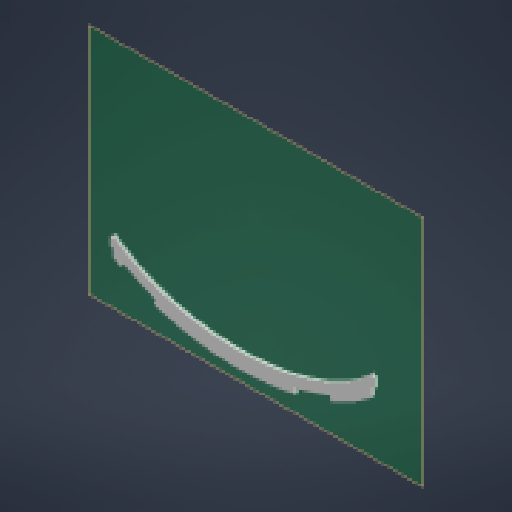
# Autodesk Inventor part: Spant
Saved by Autodesk Inventor 2023 (Build 270158000, 158)
## iProperties
Created: 2022-06-17
Part Number: Spant
Material: Generic
Document SubType Name: Modeling
Designer: bananenbrot
Density: 1 g/cm^3
Appearance: Default
Author: bananenbrot
Autodesk Inventor part; units mm, degrees
ref_plane "YZ Plane" through (0, 0, 0) normal (1, 0, 0) x (0, 1, 0)
ref_plane "XZ Plane" through (0, 0, 0) normal (0, 1, 0) x (-1, 0, 0)
ref_plane "XY Plane" through (0, 0, 0) normal (0, 0, 1) x (1, 0, 0)
ref_plane "Work Plane1" through (0, 0, 0) normal (0, 0, -1) x (-1, 0, 0)
sketch "Sketch1" plane through (0, 0, 0) normal (0, 0, -1) x (-1, 0, 0)
  spline S0 degree 3 poles (105.488254, 71.058726) (105.655909, 71.469411) (105.824043, 71.880004) (106.156862, 72.690396) (106.321597, 73.090375) (106.486681, 73.490119) knots 0 0 0 0 0.50633528 0.50633528 1 1 1 1
  spline S1 degree 3 poles (106.486681, 73.490119) (99.341384, 77.505424) (91.623026, 81.110604) (83.425971, 84.259639) knots -25.89555236 -25.89555236 -25.89555236 -25.89555236 -23.89595958 -23.89595958 -23.89595958 -23.89595958
  spline S2 degree 3 poles (83.425971, 84.259639) (83.383031, 84.186182) (83.340079, 84.112732) (83.249809, 83.958418) (83.202489, 83.877555) (83.155155, 83.796701) knots 0 0 0 0 0.47593748 0.47593748 1 1 1 1
  spline S3 degree 3 poles (83.155155, 83.796701) (82.99498, 83.50339) (82.834647, 83.210135) (82.513677, 82.623784) (82.353014, 82.330641) (82.192209, 82.037607) knots 0 0 0 0 0.49995529 0.49995529 1 1 1 1
  spline S4 degree 3 poles (82.192209, 82.037607) (86.075009, 80.386549) (89.943485, 78.66542) (97.708877, 75.024479) (101.631748, 73.086364) (105.488254, 71.058726) knots -2.57301498 -2.57301498 -2.57301498 -2.57301498 -1.30716712 -1.30716712 -0.00005006 -0.00005006 -0.00005006 -0.00005006
  spline S5 degree 3 poles (-58.922767, -91.941666) (-58.774909, -91.527729) (-58.626707, -91.113855) (-58.3286, -90.283485) (-58.17865, -89.866881) (-58.028364, -89.450461) knots 0 0 0 0 0.49821081 0.49821081 1 1 1 1
  spline S6 degree 3 poles (-58.028364, -89.450461) (-62.223821, -88.294879) (-66.410527, -87.076871) (-74.82943, -84.476914) (-79.083634, -83.084228) (-83.295327, -81.612273) knots -2.64342131 -2.64342131 -2.64342131 -2.64342131 -1.33846844 -1.33846844 -0.00001781 -0.00001781 -0.00001781 -0.00001781
  spline S7 degree 3 poles (-83.295327, -81.612273) (-83.368111, -81.939178) (-83.441155, -82.266061) (-83.587693, -82.919559) (-83.661203, -83.246243) (-83.734938, -83.572841) knots 0 0 0 0 0.50006828 0.50006828 1 1 1 1
  spline S8 degree 3 poles (-83.734938, -83.572841) (-83.752629, -83.665103) (-83.770343, -83.757362) (-83.804214, -83.933539) (-83.820367, -84.01746) (-83.836539, -84.101376) knots 0 0 0 0 0.52364207 0.52364207 1 1 1 1
  spline S9 degree 3 poles (-83.836539, -84.101376) (-75.900663, -87.170821) (-67.564129, -89.792222) (-58.922767, -91.941666) knots -18.70758966 -18.70758966 -18.70758966 -18.70758966 -16.3084011 -16.3084011 -16.3084011 -16.3084011
  spline S10 degree 3 poles (-140.156146, 42.705244) (-140.52655, 42.946666) (-140.896999, 43.188241) (-141.61629, 43.657531) (-141.965329, 43.88536) (-142.314244, 44.113207) knots 0 0 0 0 0.51480121 0.51480121 1 1 1 1
  spline S11 degree 3 poles (-142.314244, 44.113207) (-146.113734, 39.366065) (-149.438319, 34.257689) (-152.104054, 28.810883) knots -4.82793939 -4.82793939 -4.82793939 -4.82793939 -3.00658211 -3.00658211 -3.00658211 -3.00658211
  spline S12 degree 3 poles (-152.104054, 28.810883) (-152.064303, 28.781841) (-152.024554, 28.752797) (-151.909264, 28.668547) (-151.833725, 28.613333) (-151.758195, 28.558111) knots 0 0 0 0 0.344756 0.344756 1 1 1 1
  spline S13 degree 3 poles (-151.758195, 28.558111) (-151.483888, 28.367342) (-151.209569, 28.176431) (-150.661151, 27.794486) (-150.386901, 27.603345) (-150.112796, 27.412158) knots 0 0 0 0 0.49994705 0.49994705 1 1 1 1
  spline S14 degree 3 poles (-150.112796, 27.412158) (-148.553563, 30.128813) (-146.873692, 32.828621) (-143.542191, 37.897752) (-141.864648, 40.324826) (-140.156146, 42.705244) knots -1.81999292 -1.81999292 -1.81999292 -1.81999292 -0.87903361 -0.87903361 -0.00000955 -0.00000955 -0.00000955 -0.00000955
  spline S15 degree 3 poles (-55.772759, -89.028179) (-55.938485, -89.473405) (-56.103756, -89.918878) (-56.433281, -90.809909) (-56.597586, -91.255603) (-56.761424, -91.701392) knots 0 0 0 0 0.50006611 0.50006611 1 1 1 1
  spline S16 degree 3 poles (-56.761424, -91.701392) (-56.698316, -91.71797) (-56.635205, -91.734536) (-56.508995, -91.767635) (-56.445896, -91.784169) (-56.382794, -91.80069) knots 0 0 0 0 0.50007704 0.50007704 1 1 1 1
  spline S17 degree 3 poles (-56.382794, -91.80069) (-56.221993, -91.320035) (-56.060734, -90.839439) (-55.737349, -89.878637) (-55.575164, -89.398259) (-55.412537, -88.918128) knots 0 0 0 0 0.49995781 0.49995781 1 1 1 1
  spline S18 degree 3 poles (-55.412537, -88.918128) (-60.395889, -87.574654) (-65.371777, -86.143235) (-75.376216, -83.050578) (-80.443009, -81.371101) (-85.442136, -79.575514) knots -3.14153253 -3.14153253 -3.14153253 -3.14153253 -1.59354523 -1.59354523 0 0 0 0
  spline S19 degree 3 poles (-85.442136, -79.575514) (-85.600845, -80.347246) (-85.761456, -81.119077) (-86.083068, -82.648175) (-86.244205, -83.406358) (-86.406726, -84.163805) knots 0 0 0 0 0.50422346 0.50422346 1 1 1 1
  spline S20 degree 3 poles (-86.406726, -84.163805) (-90.920076, -82.353793) (-95.299024, -80.397526) (-116.019517, -70.109373) (-129.760695, -59.970512) (-146.159331, -41.459598) (-151.350121, -33.629327) (-158.207877, -17.049282) (-159.996164, -8.655283) (-159.999998, -0.018499) (-160, -0.009249) (-160, 0) knots -11.1695193 -11.1695193 -11.1695193 -11.1695193 -9.98830114 -9.98830114 -5.37837028 -5.37837028 -2.58826084 -2.58826084 0 0 0.00277479 0.00277479 0.00277479 0.00277479
  spline S21 degree 3 poles (-160, 0) (-160, 0.009249) (-159.999998, 0.018499) (-159.996164, 8.655283) (-158.207877, 17.049282) (-154.531773, 25.937027) (-154.137586, 26.837245) (-153.725914, 27.72876) knots -31.82936206 -31.82936206 -31.82936206 -31.82936206 -31.82614588 -31.82614588 -28.82616147 -28.82616147 -28.48444547 -28.48444547 -28.48444547 -28.48444547
  spline S22 degree 3 poles (-153.725914, 27.72876) (-153.133623, 27.312391) (-152.540944, 26.89493) (-151.307606, 26.024278) (-150.664927, 25.569494) (-150.024025, 25.114699) knots 0 0 0 0 0.47946727 0.47946727 1 1 1 1
  spline S23 degree 3 poles (-150.024025, 25.114699) (-148.218657, 28.38678) (-146.211118, 31.651154) (-142.262605, 37.660516) (-140.273177, 40.511906) (-138.247084, 43.294789) knots -2.15697753 -2.15697753 -2.15697753 -2.15697753 -1.03269259 -1.03269259 0 0 0 0
  spline S24 degree 3 poles (-138.247084, 43.294789) (-138.665982, 43.579459) (-139.084954, 43.86436) (-139.922388, 44.434153) (-140.341161, 44.719256) (-140.759707, 45.004364) knots 0 0 0 0 0.50002009 0.50002009 1 1 1 1
  spline S25 degree 3 poles (-140.759707, 45.004364) (-140.786159, 44.968837) (-140.812601, 44.933303) (-140.86548, 44.862206) (-140.891916, 44.826642) (-140.918342, 44.791072) knots 0 0 0 0 0.4998879 0.4998879 1 1 1 1
  spline S26 degree 3 poles (-140.918342, 44.791072) (-140.521169, 44.532497) (-140.123801, 44.273942) (-139.329134, 43.757192) (-138.931577, 43.49883) (-138.534074, 43.240669) knots 0 0 0 0 0.49997548 0.49997548 1 1 1 1
  spline S27 degree 3 poles (-138.534074, 43.240669) (-140.582745, 40.421432) (-142.593714, 37.531617) (-146.438167, 31.657619) (-148.325685, 28.585569) (-150.038777, 25.502731) knots -2.10107116 -2.10107116 -2.10107116 -2.10107116 -1.05805088 -1.05805088 0 0 0 0
  spline S28 degree 3 poles (-150.038777, 25.502731) (-150.450899, 25.794235) (-150.863559, 26.085631) (-151.688414, 26.66721) (-152.101208, 26.957814) (-152.513901, 27.247943) knots 0 0 0 0 0.50015658 0.50015658 1 1 1 1
  spline S29 degree 3 poles (-152.513901, 27.247943) (-152.715187, 27.396775) (-152.916565, 27.545554) (-153.272825, 27.808558) (-153.42774, 27.922853) (-153.582675, 28.037097) knots 0 0 0 0 0.56531165 0.56531165 1 1 1 1
  spline S30 degree 3 poles (-153.582675, 28.037097) (-150.112252, 35.463041) (-145.430604, 42.282192) (-129.760695, 59.970512) (-116.019517, 70.109373) (-76.168856, 89.89605) (-48.159301, 97.168531) (10.323594, 101.429176) (40.306692, 98.637427) (72.686621, 89.145496) (77.300324, 87.615382) (81.772002, 85.953611) knots -28.44500583 -28.44500583 -28.44500583 -28.44500583 -25.59221971 -25.59221971 -20.24897129 -20.24897129 -12.68266849 -12.68266849 -5.31702533 -5.31702533 -4.05257189 -4.05257189 -4.05257189 -4.05257189
  spline S31 degree 3 poles (81.772002, 85.953611) (81.39685, 85.277236) (81.020675, 84.601078) (80.260988, 83.24002) (79.877131, 82.554568) (79.4924, 81.86999) knots 0 0 0 0 0.49620458 0.49620458 1 1 1 1
  spline S32 degree 3 poles (79.4924, 81.86999) (84.106097, 79.944142) (88.704811, 77.920177) (97.92698, 73.597565) (102.596521, 71.267421) (107.162032, 68.805956) knots -3.05655345 -3.05655345 -3.05655345 -3.05655345 -1.55603451 -1.55603451 0 0 0 0
  spline S33 degree 3 poles (107.162032, 68.805956) (107.362525, 69.272925) (107.563697, 69.739771) (107.967009, 70.672511) (108.169269, 71.138686) (108.372016, 71.604484) knots 0 0 0 0 0.50008693 0.50008693 1 1 1 1
  spline S34 degree 3 poles (108.372016, 71.604484) (108.311413, 71.637617) (108.250793, 71.670727) (108.129563, 71.736879) (108.068966, 71.769912) (108.008356, 71.802922) knots 0 0 0 0 0.50026413 0.50026413 1 1 1 1
  spline S35 degree 3 poles (108.008356, 71.802922) (107.831652, 71.360531) (107.655471, 70.9178) (107.304315, 70.031863) (107.129254, 69.588442) (106.954875, 69.144881) knots 0 0 0 0 0.49987396 0.49987396 1 1 1 1
  spline S36 degree 3 poles (106.954875, 69.144881) (102.458096, 71.560882) (97.862015, 73.850273) (88.857802, 78.067945) (84.40815, 80.029312) (79.943507, 81.898722) knots -2.98266168 -2.98266168 -2.98266168 -2.98266168 -1.45206607 -1.45206607 0 0 0 0
  spline S37 degree 3 poles (79.943507, 81.898722) (80.189868, 82.338832) (80.435857, 82.779254) (80.926861, 83.660218) (81.171962, 84.100915) (81.416641, 84.541745) knots 0 0 0 0 0.50009335 0.50009335 1 1 1 1
  spline S38 degree 3 poles (81.416641, 84.541745) (81.544597, 84.757023) (81.672451, 84.972373) (81.922458, 85.393942) (82.044631, 85.600173) (82.166704, 85.806452) knots 0 0 0 0 0.51095751 0.51095751 1 1 1 1
  spline S39 degree 3 poles (82.166704, 85.806452) (96.340132, 80.504804) (109.079769, 73.882769) (120, 66.143783) knots -4.01533339 -4.01533339 -4.01533339 -4.01533339 0 0 0 0
  line L0 (120, 66.143783) -> (120, 64.915839)
  spline S40 degree 3 poles (120, 64.915839) (116.958046, 67.095767) (113.769602, 69.18832) (110.4451, 71.188412) knots -27.23016157 -27.23016157 -27.23016157 -27.23016157 -26.27049987 -26.27049987 -26.27049987 -26.27049987
  spline S41 degree 3 poles (110.4451, 71.188412) (110.144531, 70.479272) (109.845231, 69.769024) (109.241462, 68.327114) (108.936634, 67.594325) (108.633933, 66.86133) knots 0 0 0 0 0.49269339 0.49269339 1 1 1 1
  spline S42 degree 3 poles (108.633933, 66.86133) (103.413337, 69.741468) (98.040638, 72.443923) (87.569561, 77.343921) (82.406444, 79.594098) (77.229578, 81.721673) knots -3.46782142 -3.46782142 -3.46782142 -3.46782142 -1.67911103 -1.67911103 -0.00000822 -0.00000822 -0.00000822 -0.00000822
  spline S43 degree 3 poles (77.229578, 81.721673) (77.614353, 82.392714) (77.998129, 83.064688) (78.756084, 84.39678) (79.130603, 85.057404) (79.504014, 85.718327) knots 0 0 0 0 0.5047033 0.5047033 1 1 1 1
  spline S44 degree 3 poles (79.504014, 85.718327) (76.000382, 86.979279) (72.415021, 88.158572) (41.411665, 97.427275) (11.712347, 100.344863) (-46.584978, 96.460454) (-74.708327, 89.33117) (-114.784395, 69.723313) (-128.606876, 59.635414) (-139.39681, 47.589468) (-139.920365, 46.990667) (-140.436318, 46.385633) knots -23.57993789 -23.57993789 -23.57993789 -23.57993789 -22.74051364 -22.74051364 -16.46951252 -16.46951252 -9.96116021 -9.96116021 -5.36021524 -5.36021524 -5.12219462 -5.12219462 -5.12219462 -5.12219462
  spline S45 degree 3 poles (-140.436318, 46.385633) (-139.821337, 45.967601) (-139.205726, 45.549511) (-137.937927, 44.689331) (-137.284591, 44.246513) (-136.631622, 43.804456) knots 0 0 0 0 0.48532424 0.48532424 1 1 1 1
  spline S46 degree 3 poles (-136.631622, 43.804456) (-139.054316, 40.516338) (-141.435007, 37.123701) (-145.886157, 30.29577) (-148.055837, 26.710869) (-149.950671, 23.137939) knots -2.43253078 -2.43253078 -2.43253078 -2.43253078 -1.21332259 -1.21332259 -0.00004072 -0.00004072 -0.00004072 -0.00004072
  spline S47 degree 3 poles (-149.950671, 23.137939) (-150.579311, 23.592648) (-151.210164, 24.04715) (-152.403565, 24.90403) (-152.968317, 25.308301) (-153.532797, 25.711303) knots 0 0 0 0 0.52806556 0.52806556 1 1 1 1
  spline S48 degree 3 poles (-153.532797, 25.711303) (-153.653765, 25.431767) (-153.772984, 25.151387) (-157.199149, 16.9475) (-158.99615, 8.606573) (-158.999998, 0.018371) (-159, 0.009185) (-159, 0) knots -2.66506067 -2.66506067 -2.66506067 -2.66506067 -2.57370536 -2.57370536 0 0 0.00275564 0.00275564 0.00275564 0.00275564
  spline S49 degree 3 poles (-159, 0) (-159, -0.009185) (-158.999998, -0.018371) (-158.99615, -8.606573) (-157.199149, -16.9475) (-150.308131, -33.447912) (-145.079436, -41.245352) (-128.606876, -59.635414) (-114.784395, -69.723313) (-94.929583, -79.437598) (-91.582833, -80.947001) (-88.154881, -82.370355) knots -31.86013737 -31.86013737 -31.86013737 -31.86013737 -31.85691351 -31.85691351 -28.84590276 -28.84590276 -25.5859293 -25.5859293 -20.20322506 -20.20322506 -19.14689485 -19.14689485 -19.14689485 -19.14689485
  spline S50 degree 3 poles (-88.154881, -82.370355) (-88.005245, -81.625565) (-87.857245, -80.880017) (-87.561724, -79.371575) (-87.414116, -78.607759) (-87.268731, -77.844009) knots 0 0 0 0 0.49421065 0.49421065 1 1 1 1
  spline S51 degree 3 poles (-87.268731, -77.844009) (-81.548725, -79.948527) (-75.730398, -81.89586) (-64.370585, -85.404573) (-58.77266, -86.997837) (-53.169946, -88.480229) knots -3.56732869 -3.56732869 -3.56732869 -3.56732869 -1.7386564 -1.7386564 -0.00000461 -0.00000461 -0.00000461 -0.00000461
  spline S52 degree 3 poles (-53.169946, -88.480229) (-53.431004, -89.225816) (-53.690828, -89.9722) (-54.206068, -91.460346) (-54.461722, -92.202741) (-54.716118, -92.945222) knots 0 0 0 0 0.50162275 0.50162275 1 1 1 1
  spline S53 degree 3 poles (-54.716118, -92.945222) (-42.581047, -95.718052) (-29.888292, -97.572971) (11.712347, -100.344863) (41.411665, -97.427275) (88.330972, -83.40037) (105.768628, -75.114337) (120, -64.915839) knots -15.92125118 -15.92125118 -15.92125118 -15.92125118 -12.58902064 -12.58902064 -5.2524964 -5.2524964 0 0 0 0
  line L1 (120, -64.915839) -> (120, -66.143783)
  spline S54 degree 3 poles (120, -66.143783) (105.539645, -76.391596) (87.891779, -84.688219) (40.306692, -98.637427) (10.323594, -101.429176) (-42.625257, -97.571702) (-65.649403, -92.429988) (-85.972732, -84.337236) knots -27.4582651 -27.4582651 -27.4582651 -27.4582651 -22.87095843 -22.87095843 -16.51619015 -16.51619015 -11.20734468 -11.20734468 -11.20734468 -11.20734468
  spline S55 degree 3 poles (-85.972732, -84.337236) (-85.929472, -84.101334) (-85.886373, -83.86539) (-85.798444, -83.382085) (-85.753625, -83.134694) (-85.708998, -82.887282) knots 0 0 0 0 0.488224 0.488224 1 1 1 1
  spline S56 degree 3 poles (-85.708998, -82.887282) (-85.603052, -82.392867) (-85.49772, -81.898193) (-85.288395, -80.908503) (-85.184351, -80.41324) (-85.081049, -79.917953) knots 0 0 0 0 0.49984979 0.49984979 1 1 1 1
  spline S57 degree 3 poles (-85.081049, -79.917953) (-80.168058, -81.674386) (-75.190842, -83.31947) (-65.425689, -86.333614) (-60.603113, -87.722189) (-55.772759, -89.028179) knots -3.06681768 -3.06681768 -3.06681768 -3.06681768 -1.50113749 -1.50113749 0 0 0 0
  line L2 (-130, 140) -> (-130, -140)
  ellipse E0 centre (0, 0) end of major axis (0, -84.000351) minor radius 144 (-130, -36.129164) -> (120, -46.432941) ccw
  line L3 (120, -64.915839) -> (120, -46.432941)
  spline S58 degree 3 poles (83.155155, -83.796701) (83.202489, -83.877556) (83.24981, -83.958419) (83.340079, -84.112732) (83.383031, -84.186182) (83.425971, -84.259639) knots 0 0 0 0 0.52406443 0.52406443 1 1 1 1
  spline S59 degree 3 poles (83.425971, -84.259639) (91.623023, -81.110605) (99.341382, -77.505425) (106.486681, -73.490119) knots -3.90072545 -3.90072545 -3.90072545 -3.90072545 -1.56137635 -1.56137635 -1.56137635 -1.56137635
  spline S60 degree 3 poles (106.486681, -73.490119) (106.321618, -73.090425) (106.156903, -72.690495) (105.824083, -71.880103) (105.655929, -71.469461) (105.488254, -71.058726) knots 0 0 0 0 0.49360341 0.49360341 1 1 1 1
  spline S61 degree 3 poles (105.488254, -71.058726) (101.601392, -73.102325) (97.647003, -75.055044) (89.880457, -78.693455) (86.043436, -80.399975) (82.192209, -82.037607) knots -2.57282162 -2.57282162 -2.57282162 -2.57282162 -1.25548991 -1.25548991 -0.00000561 -0.00000561 -0.00000561 -0.00000561
  spline S62 degree 3 poles (82.192209, -82.037607) (82.353014, -82.330641) (82.513677, -82.623785) (82.834648, -83.210136) (82.99498, -83.50339) (83.155155, -83.796701) knots 0 0 0 0 0.50004508 0.50004508 1 1 1 1
  spline S63 degree 3 poles (-58.028364, -89.450461) (-62.233064, -88.292333) (-66.429007, -87.071495) (-74.847725, -84.470924) (-79.092678, -83.081067) (-83.295327, -81.612273) knots -2.64341286 -2.64341286 -2.64341286 -2.64341286 -1.33558505 -1.33558505 -0.00000826 -0.00000826 -0.00000826 -0.00000826
  spline S64 degree 3 poles (-83.295327, -81.612273) (-83.368111, -81.939178) (-83.441155, -82.266061) (-83.587693, -82.91956) (-83.661203, -83.246244) (-83.734938, -83.572841) knots 0 0 0 0 0.50006844 0.50006844 1 1 1 1
  spline S65 degree 3 poles (-83.734938, -83.572841) (-83.752651, -83.665214) (-83.770386, -83.757584) (-83.804257, -83.933762) (-83.820388, -84.017571) (-83.836539, -84.101376) knots 0 0 0 0 0.52427325 0.52427325 1 1 1 1
  spline S66 degree 3 poles (-83.836539, -84.101376) (-77.593042, -86.516243) (-71.077682, -88.662135) (-64.355901, -90.51692) (-62.559229, -91.012688) (-60.747638, -91.487388) (-58.922767, -91.941666) knots 0 0 0 0 0.78908463 0.78908463 0.78908463 1 1 1 1
  spline S67 degree 3 poles (-58.922767, -91.941666) (-58.774903, -91.527713) (-58.626695, -91.113822) (-58.328588, -90.283452) (-58.178644, -89.866865) (-58.028364, -89.450461) knots 0 0 0 0 0.49823074 0.49823074 1 1 1 1
  spline S68 degree 3 poles (82.192209, 82.037607) (86.086099, 80.381833) (89.965626, 78.655569) (97.730611, 75.013739) (101.642413, 73.080757) (105.488254, 71.058726) knots -2.57298365 -2.57298365 -2.57298365 -2.57298365 -1.3035202 -1.3035202 -0.00001762 -0.00001762 -0.00001762 -0.00001762
  spline S69 degree 3 poles (105.488254, 71.058726) (105.65593, 71.469462) (105.824085, 71.880106) (106.156904, 72.690498) (106.321618, 73.090426) (106.486681, 73.490119) knots 0 0 0 0 0.50639849 0.50639849 1 1 1 1
  spline S70 degree 3 poles (106.486681, 73.490119) (99.336447, 77.508199) (91.617269, 81.112815) (83.425971, 84.259639) knots -20.48335777 -20.48335777 -20.48335777 -20.48335777 -18.34027175 -18.34027175 -18.34027175 -18.34027175
  spline S71 degree 3 poles (83.425971, 84.259639) (83.383031, 84.186182) (83.340079, 84.112732) (83.249809, 83.958418) (83.202489, 83.877555) (83.155155, 83.796701) knots 0 0 0 0 0.4759375 0.4759375 1 1 1 1
  spline S72 degree 3 poles (83.155155, 83.796701) (82.99498, 83.50339) (82.834647, 83.210135) (82.513677, 82.623784) (82.353014, 82.330641) (82.192209, 82.037607) knots 0 0 0 0 0.49995542 0.49995542 1 1 1 1
  spline S73 degree 3 poles (-83.295327, 81.612273) (-79.056214, 83.093811) (-74.773955, 84.495073) (-66.354492, 87.093168) (-62.195794, 88.302599) (-58.028364, 89.450461) knots -2.64454735 -2.64454735 -2.64454735 -2.64454735 -1.29681005 -1.29681005 -0.00002349 -0.00002349 -0.00002349 -0.00002349
  spline S74 degree 3 poles (-58.028364, 89.450461) (-58.178669, 89.866933) (-58.328637, 90.283589) (-58.626744, 91.113959) (-58.774927, 91.527781) (-58.922767, 91.941666) knots 0 0 0 0 0.50185207 0.50185207 1 1 1 1
  spline S75 degree 3 poles (-58.922767, 91.941666) (-67.552935, 89.794994) (-75.890466, 87.174767) (-83.836539, 84.101376) knots -7.08866348 -7.08866348 -7.08866348 -7.08866348 -4.92689897 -4.92689897 -4.92689897 -4.92689897
  spline S76 degree 3 poles (-83.836539, 84.101376) (-83.820367, 84.01746) (-83.804214, 83.93354) (-83.770343, 83.757363) (-83.752629, 83.665103) (-83.734938, 83.572841) knots 0 0 0 0 0.47635613 0.47635613 1 1 1 1
  spline S77 degree 3 poles (-83.734938, 83.572841) (-83.661203, 83.246243) (-83.587693, 82.919559) (-83.441155, 82.26606) (-83.368111, 81.939178) (-83.295327, 81.612273) knots 0 0 0 0 0.49993221 0.49993221 1 1 1 1
  spline S78 degree 3 poles (120, 64.915839) (116.957002, 67.096515) (113.76848, 69.188995) (110.4451, 71.188412) knots -21.91218991 -21.91218991 -21.91218991 -21.91218991 -20.88499187 -20.88499187 -20.88499187 -20.88499187
  spline S79 degree 3 poles (110.4451, 71.188412) (110.14453, 70.479268) (109.845229, 69.769017) (109.241459, 68.327108) (108.936633, 67.594322) (108.633933, 66.86133) knots 0 0 0 0 0.49269556 0.49269556 1 1 1 1
  spline S80 degree 3 poles (108.633933, 66.86133) (103.399335, 69.749193) (98.011719, 72.458471) (87.539917, 77.356836) (82.391633, 79.600185) (77.229578, 81.721673) knots -3.46781506 -3.46781506 -3.46781506 -3.46781506 -1.67430729 -1.67430729 -0.00000822 -0.00000822 -0.00000822 -0.00000822
  spline S81 degree 3 poles (77.229578, 81.721673) (77.614354, 82.392716) (77.998131, 83.064691) (78.756086, 84.396783) (79.130604, 85.057405) (79.504014, 85.718327) knots 0 0 0 0 0.5047044 0.5047044 1 1 1 1
  spline S82 degree 3 poles (79.504014, 85.718327) (73.308954, 87.94792) (66.861755, 89.921003) (36.694093, 97.614716) (11.758891, 99.889296) (-27.015369, 97.977443) (-41.19803, 96.03407) (-54.716118, 92.945222) knots -18.00144011 -18.00144011 -18.00144011 -18.00144011 -16.40919862 -16.40919862 -10.78869968 -10.78869968 -7.43834932 -7.43834932 -7.43834932 -7.43834932
  spline S83 degree 3 poles (-54.716118, 92.945222) (-54.461721, 92.202737) (-54.206066, 91.460338) (-53.690825, 89.972192) (-53.431002, 89.225812) (-53.169946, 88.480229) knots 0 0 0 0 0.49837992 0.49837992 1 1 1 1
  spline S84 degree 3 poles (-53.169946, 88.480229) (-58.845945, 86.978447) (-64.517386, 85.362779) (-75.875221, 81.847348) (-81.619734, 79.922402) (-87.268731, 77.844009) knots -3.5669406 -3.5669406 -3.5669406 -3.5669406 -1.80576616 -1.80576616 -0.00000315 -0.00000315 -0.00000315 -0.00000315
  spline S85 degree 3 poles (-87.268731, 77.844009) (-87.414117, 78.607768) (-87.561728, 79.371592) (-87.857248, 80.880034) (-88.005246, 81.625573) (-88.154881, 82.370355) knots 0 0 0 0 0.50579491 0.50579491 1 1 1 1
  spline S86 degree 3 poles (-88.154881, 82.370355) (-104.503687, 75.582004) (-118.684509, 66.972452) (-130, 56.965589) knots -4.53204805 -4.53204805 -4.53204805 -4.53204805 -0.00045691 -0.00045691 -0.00045691 -0.00045691
  line L4 (-130, 56.965589) -> (-130, 58.296119)
  spline S87 degree 3 poles (-130, 58.296119) (-118.207585, 68.568391) (-103.411704, 77.344214) (-86.406726, 84.163805) knots -23.34438249 -23.34438249 -23.34438249 -23.34438249 -18.59383478 -18.59383478 -18.59383478 -18.59383478
  spline S88 degree 3 poles (-86.406726, 84.163805) (-86.244204, 83.406352) (-86.083065, 82.648162) (-85.761453, 81.119064) (-85.600844, 80.347239) (-85.442136, 79.575514) knots 0 0 0 0 0.49578079 0.49578079 1 1 1 1
  spline S89 degree 3 poles (-85.442136, 79.575514) (-80.397499, 81.387447) (-75.283769, 83.081215) (-65.278219, 86.170137) (-60.349134, 87.587259) (-55.412537, 88.918128) knots -3.14230865 -3.14230865 -3.14230865 -3.14230865 -1.53385404 -1.53385404 0 0 0 0
  spline S90 degree 3 poles (-55.412537, 88.918128) (-55.575164, 89.39826) (-55.737349, 89.878639) (-56.060735, 90.839441) (-56.221993, 91.320036) (-56.382794, 91.80069) knots 0 0 0 0 0.50004299 0.50004299 1 1 1 1
  spline S91 degree 3 poles (-56.382794, 91.80069) (-56.445896, 91.784169) (-56.508995, 91.767635) (-56.635205, 91.734536) (-56.698317, 91.71797) (-56.761424, 91.701392) knots 0 0 0 0 0.49992367 0.49992367 1 1 1 1
  spline S92 degree 3 poles (-56.761424, 91.701392) (-56.597585, 91.255602) (-56.43328, 90.809907) (-56.103755, 89.918876) (-55.938485, 89.473404) (-55.772759, 89.028179) knots 0 0 0 0 0.49993492 0.49993492 1 1 1 1
  spline S93 degree 3 poles (-55.772759, 89.028179) (-60.650289, 87.709433) (-65.520078, 86.306431) (-75.284135, 83.288618) (-80.214017, 81.657955) (-85.081049, 79.917953) knots -3.06599686 -3.06599686 -3.06599686 -3.06599686 -1.55061421 -1.55061421 0 0 0 0
  spline S94 degree 3 poles (-85.081049, 79.917953) (-85.184352, 80.413241) (-85.288396, 80.908506) (-85.49772, 81.898196) (-85.603052, 82.392868) (-85.708998, 82.887282) knots 0 0 0 0 0.50015183 0.50015183 1 1 1 1
  spline S95 degree 3 poles (-85.708998, 82.887282) (-85.753625, 83.134694) (-85.798444, 83.382086) (-85.886373, 83.865391) (-85.929472, 84.101334) (-85.972732, 84.337236) knots 0 0 0 0 0.51177654 0.51177654 1 1 1 1
  spline S96 degree 3 poles (-85.972732, 84.337236) (-84.39827, 84.964186) (-82.805012, 85.574409) (-61.249176, 93.508605) (-39.799713, 97.77755) (10.323594, 101.429176) (40.306692, 98.637427) (72.686621, 89.145496) (77.300324, 87.615382) (81.772002, 85.953611) knots -18.55346544 -18.55346544 -18.55346544 -18.55346544 -18.11458791 -18.11458791 -12.68266849 -12.68266849 -5.31702533 -5.31702533 -4.05257189 -4.05257189 -4.05257189 -4.05257189
  spline S97 degree 3 poles (81.772002, 85.953611) (81.396849, 85.277235) (81.020673, 84.601075) (80.260986, 83.240017) (79.87713, 82.554567) (79.4924, 81.86999) knots 0 0 0 0 0.49620556 0.49620556 1 1 1 1
  spline S98 degree 3 poles (79.4924, 81.86999) (84.123686, 79.9368) (88.73997, 77.904703) (97.961374, 73.580395) (102.613292, 71.258379) (107.162032, 68.805956) knots -3.05655776 -3.05655776 -3.05655776 -3.05655776 -1.55031837 -1.55031837 0 0 0 0
  spline S99 degree 3 poles (107.162032, 68.805956) (107.362525, 69.272925) (107.563698, 69.739772) (107.967009, 70.672512) (108.169269, 71.138686) (108.372016, 71.604484) knots 0 0 0 0 0.50008746 0.50008746 1 1 1 1
  spline S100 degree 3 poles (108.372016, 71.604484) (108.311413, 71.637617) (108.250793, 71.670727) (108.129563, 71.736879) (108.068966, 71.769913) (108.008356, 71.802922) knots 0 0 0 0 0.50026455 0.50026455 1 1 1 1
  spline S101 degree 3 poles (108.008356, 71.802922) (107.831651, 71.360531) (107.655471, 70.917799) (107.304314, 70.031862) (107.129254, 69.588442) (106.954875, 69.144881) knots 0 0 0 0 0.49987468 0.49987468 1 1 1 1
  spline S102 degree 3 poles (106.954875, 69.144881) (102.448301, 71.566144) (97.841942, 73.860273) (88.837298, 78.076982) (84.397889, 80.033608) (79.943507, 81.898722) knots -2.98265816 -2.98265816 -2.98265816 -2.98265816 -1.44872878 -1.44872878 0 0 0 0
  spline S103 degree 3 poles (79.943507, 81.898722) (80.189868, 82.338833) (80.435857, 82.779254) (80.926861, 83.660218) (81.171962, 84.100915) (81.416641, 84.541745) knots 0 0 0 0 0.5000937 0.5000937 1 1 1 1
  spline S104 degree 3 poles (81.416641, 84.541745) (81.544597, 84.757023) (81.672451, 84.972373) (81.922459, 85.393942) (82.044631, 85.600173) (82.166704, 85.806452) knots 0 0 0 0 0.51095765 0.51095765 1 1 1 1
  spline S105 degree 3 poles (82.166704, 85.806452) (96.340127, 80.504806) (109.079769, 73.882769) (120, 66.143783) knots -4.01533339 -4.01533339 -4.01533339 -4.01533339 0 0 0 0
  line L5 (120, 66.143783) -> (120, 64.915839)
  spline S106 degree 3 poles (-56.761424, -91.701392) (-56.698316, -91.717971) (-56.635205, -91.734536) (-56.508995, -91.767635) (-56.445896, -91.784169) (-56.382794, -91.80069) knots 0 0 0 0 0.50007725 0.50007725 1 1 1 1
  spline S107 degree 3 poles (-56.382794, -91.80069) (-56.221993, -91.320035) (-56.060734, -90.839439) (-55.737349, -89.878637) (-55.575164, -89.398259) (-55.412537, -88.918128) knots 0 0 0 0 0.49995803 0.49995803 1 1 1 1
  spline S108 degree 3 poles (-55.412537, -88.918128) (-60.410207, -87.570794) (-65.400429, -86.134993) (-75.404526, -83.041192) (-80.456947, -81.366095) (-85.442136, -79.575514) knots -3.14153527 -3.14153527 -3.14153527 -3.14153527 -1.58910232 -1.58910232 0 0 0 0
  spline S109 degree 3 poles (-85.442136, -79.575514) (-85.600846, -80.347247) (-85.761456, -81.119081) (-86.083069, -82.648179) (-86.244206, -83.40636) (-86.406726, -84.163805) knots 0 0 0 0 0.50422465 0.50422465 1 1 1 1
  ellipse E1 centre (0, 0) end of major axis (160, 0) minor radius 100 (-130, -58.296119) -> (-86.406726, -84.163805) ccw
  line L6 (-130, -58.296119) -> (-130, -56.965589)
  spline S110 degree 3 poles (-130, -56.965589) (-125.622291, -60.837019) (-120.7953, -64.515531) (-115.568661, -67.961571) (-107.344581, -73.38389) (-98.127989, -78.229321) (-88.154881, -82.370355) knots 0 0 0 0 0.38857691 0.38857691 0.38857691 1 1 1 1
  spline S111 degree 3 poles (-88.154881, -82.370355) (-88.005261, -81.625648) (-87.857277, -80.880183) (-87.561756, -79.371741) (-87.414132, -78.607842) (-87.268731, -77.844009) knots 0 0 0 0 0.49415576 0.49415576 1 1 1 1
  spline S112 degree 3 poles (-87.268731, -77.844009) (-81.53492, -79.953606) (-75.702237, -81.905287) (-64.342042, -85.412695) (-58.758411, -87.001607) (-53.169946, -88.480229) knots -3.56731676 -3.56731676 -3.56731676 -3.56731676 -1.73423435 -1.73423435 -0.00000461 -0.00000461 -0.00000461 -0.00000461
  spline S113 degree 3 poles (-53.169946, -88.480229) (-53.431002, -89.22581) (-53.690824, -89.972189) (-54.206064, -91.460335) (-54.46172, -92.202735) (-54.716118, -92.945222) knots 0 0 0 0 0.50161891 0.50161891 1 1 1 1
  spline S114 degree 3 poles (-54.716118, -92.945222) (-37.103886, -96.969571) (-18.340613, -99.030517) (0.419495, -98.999655) (23.518657, -98.961655) (46.590543, -95.73532) (67.499159, -89.624011) (71.587609, -88.429012) (75.592712, -87.124235) (79.504014, -85.718327) knots -1.92129687 -1.92129687 -1.92129687 -1.92129687 -1.5681642 -1.5681642 -1.5681642 -1.13335493 -1.13335493 -1.13335493 -1.04833277 -1.04833277 -1.04833277 -1.04833277
  spline S115 degree 3 poles (79.504014, -85.718327) (79.130601, -85.057399) (78.756078, -84.39677) (77.998123, -83.064678) (77.61435, -82.392709) (77.229578, -81.721673) knots 0 0 0 0 0.49530047 0.49530047 1 1 1 1
  spline S116 degree 3 poles (77.229578, -81.721673) (82.493633, -79.558265) (87.744095, -77.267835) (98.210861, -72.358213) (103.495791, -69.695979) (108.633933, -66.86133) knots -3.46785791 -3.46785791 -3.46785791 -3.46785791 -1.76047655 -1.76047655 -0.00001749 -0.00001749 -0.00001749 -0.00001749
  spline S117 degree 3 poles (108.633933, -66.86133) (108.936639, -67.594336) (109.24147, -68.327135) (109.84524, -69.769045) (110.144536, -70.479282) (110.4451, -71.188412) knots 0 0 0 0 0.50731401 0.50731401 1 1 1 1
  spline S118 degree 3 poles (110.4451, -71.188412) (113.769602, -69.18832) (116.958046, -67.095767) (120, -64.915839) knots -1.12272047 -1.12272047 -1.12272047 -1.12272047 0 0 0 0
  line L7 (120, -64.915839) -> (120, -66.143783)
  spline S119 degree 3 poles (120, -66.143783) (109.056689, -73.899126) (96.285436, -80.525263) (82.166705, -85.806452) knots -21.95297363 -21.95297363 -21.95297363 -21.95297363 -18.27712891 -18.27712891 -18.27712891 -18.27712891
  spline S120 degree 3 poles (82.166705, -85.806452) (82.044631, -85.600172) (81.922458, -85.393942) (81.672451, -84.972373) (81.544597, -84.757023) (81.416641, -84.541745) knots 0 0 0 0 0.48904289 0.48904289 1 1 1 1
  spline S121 degree 3 poles (81.416641, -84.541745) (81.171961, -84.100914) (80.92686, -83.660215) (80.435856, -82.779252) (80.189868, -82.338831) (79.943507, -81.898722) knots 0 0 0 0 0.49990784 0.49990784 1 1 1 1
  spline S122 degree 3 poles (79.943507, -81.898722) (84.46361, -80.00609) (88.968632, -78.019084) (97.970501, -73.796201) (102.511041, -71.532436) (106.954875, -69.144881) knots -2.98427203 -2.98427203 -2.98427203 -2.98427203 -1.51338261 -1.51338261 0 0 0 0
  spline S123 degree 3 poles (106.954875, -69.144881) (107.129255, -69.588445) (107.304316, -70.031867) (107.655473, -70.917805) (107.831653, -71.360534) (108.008356, -71.802922) knots 0 0 0 0 0.50012853 0.50012853 1 1 1 1
  spline S124 degree 3 poles (108.008356, -71.802922) (108.068966, -71.769912) (108.129563, -71.736878) (108.250794, -71.670727) (108.311413, -71.637617) (108.372016, -71.604484) knots 0 0 0 0 0.49973733 0.49973733 1 1 1 1
  spline S125 degree 3 poles (108.372016, -71.604484) (108.169268, -71.138684) (107.967007, -70.672507) (107.563696, -69.739767) (107.362524, -69.272923) (107.162032, -68.805956) knots 0 0 0 0 0.49991524 0.49991524 1 1 1 1
  spline S126 degree 3 poles (107.162032, -68.805956) (102.546098, -71.294606) (97.823548, -73.649166) (88.599094, -77.966684) (84.053207, -79.96622) (79.4924, -81.86999) knots -3.05517932 -3.05517932 -3.05517932 -3.05517932 -1.48265878 -1.48265878 0 0 0 0
  spline S127 degree 3 poles (79.4924, -81.86999) (79.877133, -82.554572) (80.260992, -83.240027) (81.020679, -84.601086) (81.396852, -85.27724) (81.772002, -85.953611) knots 0 0 0 0 0.50379827 0.50379827 1 1 1 1
  ellipse E2 centre (0, 0) end of major axis (160, 0) minor radius 100 (-85.972732, -84.337236) -> (81.772002, -85.953611) ccw
  spline S128 degree 3 poles (-85.972732, -84.337236) (-85.929472, -84.101334) (-85.886373, -83.86539) (-85.798444, -83.382085) (-85.753625, -83.134694) (-85.708998, -82.887282) knots 0 0 0 0 0.48822419 0.48822419 1 1 1 1
  spline S129 degree 3 poles (-85.708998, -82.887282) (-85.603052, -82.392866) (-85.49772, -81.898192) (-85.288395, -80.908502) (-85.184351, -80.413239) (-85.081049, -79.917953) knots 0 0 0 0 0.49985033 0.49985033 1 1 1 1
  spline S130 degree 3 poles (-85.081049, -79.917953) (-80.15855, -81.677785) (-75.171541, -83.32585) (-65.406162, -86.339235) (-60.593352, -87.724828) (-55.772759, -89.028179) knots -3.06681307 -3.06681307 -3.06681307 -3.06681307 -1.49810422 -1.49810422 0 0 0 0
  spline S131 degree 3 poles (-55.772759, -89.028179) (-55.938485, -89.473405) (-56.103756, -89.918878) (-56.433281, -90.80991) (-56.597586, -91.255603) (-56.761424, -91.701392) knots 0 0 0 0 0.50006637 0.50006637 1 1 1 1
  point P0 (-144, 0)
  point P1 (0.001352, -84.000351)
  point P2 (0.001352, -99.000351)
  point P3 (-130, -56.96558)
  point P4 (-130, -56.965589)
  point P5 (110.445093, -71.188396)
  dimension "d0" = 15
  dimension "d1" = 15
  constraints: 16 end point, 8 vertical, 1 coincident, 1 horizontal alignment, 1 point on line, 1 vertical alignment, 506 other
  measures "d0" distance of point (-159, 0) point (-144, 0)
  measures "d1" distance of point (0.001, -84) point (0.001, -99)
sketch "Sketch1 outline for Extrusion1" plane through (0, 0, 0) normal (0, 0, -1) x (-1, 0, 0)
  spline S0 degree 2 poles (-130, -36.129164) (-20.600041, -170.07827) (120, -46.432941) knots 0 0 0 1 1 1 weights 1 0.49266415 1
  line L0 (120, -64.915839) -> (120, -46.432941)
  spline S1 degree 3 poles (110.445093, -71.188396) (113.769601, -69.188315) (116.958047, -67.095767) (120, -64.915839) knots 0 0 0 0 1 1 1 1
  spline S2 degree 3 poles (108.633933, -66.86133) (108.936639, -67.594336) (109.24147, -68.327135) (109.845238, -69.76904) (110.144531, -70.479271) (110.445093, -71.188396) knots 0 0 0 0 0.50731592 0.50731592 1 1 1 1
  spline S3 degree 3 poles (77.229578, -81.721673) (82.493633, -79.558265) (87.744095, -77.267835) (98.210861, -72.358213) (103.495791, -69.695979) (108.633933, -66.86133) knots 0 0 0 0 0.49234716 0.49234716 1 1 1 1
  spline S4 degree 3 poles (79.504014, -85.718327) (79.130601, -85.057399) (78.756078, -84.39677) (77.998123, -83.064678) (77.61435, -82.392709) (77.229578, -81.721673) knots 0 0 0 0 0.49530047 0.49530047 1 1 1 1
  spline S5 degree 3 poles (-54.716118, -92.945222) (-37.103886, -96.969571) (-18.340613, -99.030517) (0.419495, -98.999655) (23.518657, -98.961655) (46.590543, -95.73532) (67.499159, -89.624011) (71.587609, -88.429012) (75.592712, -87.124235) (79.504014, -85.718327) knots 0 0 0 0 0.40452141 0.40452141 0.40452141 0.9026052 0.9026052 0.9026052 1 1 1 1
  spline S6 degree 3 poles (-53.169946, -88.480229) (-53.431004, -89.225816) (-53.690828, -89.9722) (-54.206068, -91.460346) (-54.461722, -92.202741) (-54.716118, -92.945222) knots 0 0 0 0 0.50162275 0.50162275 1 1 1 1
  spline S7 degree 3 poles (-87.268731, -77.844009) (-81.548725, -79.948527) (-75.730398, -81.89586) (-64.370585, -85.404573) (-58.77266, -86.997837) (-53.169946, -88.480229) knots 0 0 0 0 0.51261737 0.51261737 1 1 1 1
  spline S8 degree 3 poles (-88.154881, -82.370355) (-88.005245, -81.625565) (-87.857245, -80.880017) (-87.561724, -79.371575) (-87.414116, -78.607759) (-87.268731, -77.844009) knots 0 0 0 0 0.49421065 0.49421065 1 1 1 1
  spline S9 degree 3 poles (-130, -56.965589) (-125.622291, -60.837019) (-120.7953, -64.515531) (-115.568661, -67.961571) (-107.344581, -73.38389) (-98.127989, -78.229321) (-88.154881, -82.370355) knots 0 0 0 0 0.38857691 0.38857691 0.38857691 1 1 1 1
  line L1 (-130, -36.129164) -> (-130, -56.965589)
extrude "Extrusion1" add sketch "Sketch1 outline for Extrusion1" along normal mid plane 3
sketch "Sketch2" plane through (0, 0, 1.5) normal (0, 0, 1) x (1, 0, 0)
  line L0 (-117, -59.67439) -> (-120, -59.67439)
  line L1 (-120, -59.67439) -> (-120, -51.67439)
  line L2 (-120, -51.67439) -> (-117, -51.67439)
  line L3 (-117, -51.67439) -> (-117, -59.67439)
  line L4 (-120, -46.432941) -> (-120, -64.915839)
  line L5 (-117, -71.406989) -> (-128.579566, -71.406989)
  line L6 (-117, -59.67439) -> (-120, -59.67439)
  line L7 (-120, -59.67439) -> (-120, -69.598951)
  line L8 (-120, -69.598951) -> (-117, -69.598951)
  line L9 (-117, -69.598951) -> (-117, -59.67439)
  line L10 (-117, -51.67439) -> (-120, -51.67439)
  line L11 (-120, -51.67439) -> (-120, -38.152806)
  line L12 (-120, -38.152806) -> (-117, -38.152806)
  line L13 (-117, -38.152806) -> (-117, -51.67439)
  point P0 (0, 0)
  point P1 (-120, -55.67439)
  point P2 (-120, -51.67439)
  point P3 (-120, -59.67439)
  point P4 (-120, -64.915839)
  dimension "d4" = 3
  dimension "d5" = 8
  constraints: 26 end point, 6 parallel, 3 horizontal, 3 perpendicular, 2 midpoint, 1 point on line
  measures "d4" distance of L0.start L0.end
  measures "d5" distance of L2.end L0.start
extrude "Extrusion2" cut sketch "Sketch2" against normal blind 3 contours L9 L8 L7 L4 L0 | L2 L4 L11 L12 L13
sketch "Sketch3" plane through (0, 0, 1.5) normal (0, 0, 1) x (1, 0, 0)
  line L0 (130, -42.547372) -> (127, -42.547372)
  line L1 (127, -42.547372) -> (127, -50.547372)
  line L2 (127, -50.547372) -> (130, -50.547372)
  line L3 (130, -50.547372) -> (130, -42.547372)
  line L4 (130, -56.96558) -> (130, -36.129164)
  line L5 (127, -50.547372) -> (130, -50.547372)
  line L6 (130, -50.547372) -> (130, -68.488731)
  line L7 (130, -68.488731) -> (127, -68.488731)
  line L8 (127, -68.488731) -> (127, -50.547372)
  line L9 (127, -42.547372) -> (130, -42.547372)
  line L10 (130, -42.547372) -> (130, -28.365328)
  line L11 (130, -28.365328) -> (127, -28.365328)
  line L12 (127, -28.365328) -> (127, -42.547372)
  point P0 (0, 0)
  point P1 (130, -46.547372)
  dimension "d8" = 8
  dimension "d9" = 3
  constraints: 24 end point, 6 parallel, 3 horizontal, 3 perpendicular, 2 midpoint, 1 point on line
  measures "d8" distance of L0.end L1.end
  measures "d9" distance of L1.end L2.end
extrude "Extrusion3" cut sketch "Sketch3" against normal blind 3 contours L0 L12 L11 L10 L4 | L4 L6 L7 L8 L2
body "Solid1"
